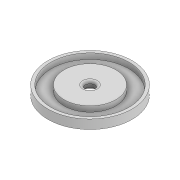
# Autodesk Inventor part: Cap V2 (App V5)
Saved by Autodesk Inventor 2021.3 (Build 253353000, 353)
## iProperties
Created: 2022-06-29
Part Number: Cap V2 (App V5)
Material: Generic
Document SubType Name: Modeling
Designer: david
Density: 1 g/cm^3
Appearance: Default
Author: david
Autodesk Inventor part; units mm, degrees
ref_plane "YZ Plane" through (0, 0, 0) normal (1, 0, 0) x (0, 1, 0)
ref_plane "XZ Plane" through (0, 0, 0) normal (0, 1, 0) x (-1, 0, 0)
ref_plane "XY Plane" through (0, 0, 0) normal (0, 0, 1) x (1, 0, 0)
sketch "Sketch1" plane through (0, 0, 0) normal (0, 1, 0) x (-1, 0, 0)
  circle A0 centre (0, 0) radius 21.35
  circle A1 centre (0, 0) radius 14.25
  circle A2 centre (0, 0) radius 23.15
  dimension "d0" = 42.7
  dimension "d1" = 28.5
  dimension "d3" = 1.8
  constraints: 3 centre point, 3 coincident
  measures "d0" diameter of A0
  measures "d1" diameter of A1
  measures "d3" radial gap between concentric circles of A2 A0
extrude "Extrusion1" add sketch "Sketch1" along normal blind 5
extrude "Extrusion2" add sketch "Sketch1" along normal blind 2 contours A0
draft "FaceDraft1" angle 3.3 pull direction (0, 1, 0) faces at (-21.0735, 4, -3.4248) fixed edges at (21.35, 2, 0)
hole "Hole1" at (0, 0, 0) direction (0, 1, 0) diameter 5.3 end through all
chamfer "Chamfer1" distance 2 angle 45 1 edges at (0, 0, 2.65)
fillet "Fillet1" radius 1.4 1 edges at (0, 5, 2.65)
body "Solid1"
